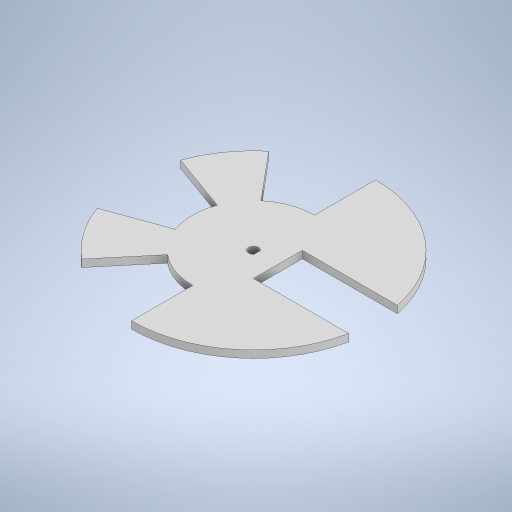
# Autodesk Inventor part: rolling_plate_small
Saved by Autodesk Inventor 2024 (Build 280153000, 153)
## iProperties
Created: 2024-04-09
Part Number: rolling_plate_small
Material: 一般
Document SubType Name: Modeling
Designer: USER
Density: 1 g/cm^3
Appearance: 預設
Author: USER
Autodesk Inventor part; units mm, degrees
ref_plane "YZ Plane" through (0, 0, 0) normal (1, 0, 0) x (0, 1, 0)
ref_plane "XZ Plane" through (0, 0, 0) normal (0, 1, 0) x (-1, 0, 0)
ref_plane "XY Plane" through (0, 0, 0) normal (0, 0, 1) x (1, 0, 0)
sketch "草圖1" plane through (0, 0, 0) normal (0, 1, 0) x (-1, 0, 0)
  circle A0 centre (0, 0) radius 50
  circle A1 centre (0, 0) radius 25
  line L0 (-50, 10) -> (-10, 10)
  line L1 (-10, 10) -> (-10, -10)
  line L2 (-10, -10) -> (-50, -10)
  line L3 (-50, -10) -> (-50, 10)
  line L4 (0, 0) -> (0, -50)
  line L5 (0, 0) -> (32.1394, -38.3022)
  arc A2 (0, -50) -> (32.1394, -38.3022) centre (0, 0) ccw
  line L6 (0, 0) -> (46.9846, -17.101)
  line L7 (0, 0) -> (46.9846, 17.101)
  arc A3 (46.9846, -17.101) -> (46.9846, 17.101) centre (0, 0) ccw
  line L8 (0, 0) -> (32.1394, 38.3022)
  line L9 (0, 0) -> (0, 50)
  arc A4 (32.1394, 38.3022) -> (0, 50) centre (0, 0) ccw
  circle A5 centre (0, 0) radius 2
  line L10 (-1.5, 1.3229) -> (-1.5, -1.3229)
  point P0 (16.0697, -19.1511)
  point P1 (0, -25)
  point P2 (-48.9898, 10)
  point P3 (-48.9898, -10)
  point P4 (16.0697, 19.1511)
  point P5 (0, 25)
  point P6 (23.4923, -8.5505)
  point P7 (23.4923, 8.5505)
  point P8 (-50, 0)
  dimension "d0" = 100
  dimension "d1" = 50
  dimension "d2" = 20
  dimension "d3" = 40
  dimension "d5" = 40
  dimension "d6" = 50
  dimension "d9" = 140
  dimension "d28" = 4
  dimension "d29" = 1.5
  dimension "d30" = 50
  constraints: 22 end point, 8 point on circle, 6 coincident, 5 centre point, 3 point on line, 2 parallel, 2 vertical, 1 horizontal, 1 horizontal alignment, 1 midpoint, 1 perpendicular, 20 other
  measures "d1" diameter of A1
  measures "d2" distance of L2.end L0.start
  measures "d3" distance of L1.end L2.end
  measures "d5" angle of L4 L5
  measures "d6" distance of L4.start L5.end
  measures "d28" diameter of A5
  measures "d29" distance between parallel lines of L4 L10
  measures "d30" radius of A2
extrude "擠出1" add sketch "草圖1" along normal blind 3 contours L7 A1 L8 A0 | A0 L5 A1 L6 | L7 A5 L8 A1 | A1 L6 A5 L7 | A1 L5 A5 L6 | L9 A1 L0 A0 | L8 A5 L9 A1 | A0 L2 A1 L4 | A1 L4 A5 L5 | L9 A5 L4 A1 L2 L1 L0 | L10 A5
